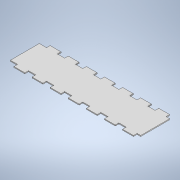
# Autodesk Inventor part: BridgeRoof
Saved by Autodesk Inventor 2022 (Build 260153000, 153)
## iProperties
Created: 2022-03-02
Part Number: BridgeRoof
Material: Generic
Document SubType Name: Modeling
Designer: anjarwala7025
Density: 1 g/cm^3
Appearance: Default
Author: anjarwala7025
Autodesk Inventor part; units mm, degrees
ref_plane "YZ Plane" through (0, 0, 0) normal (1, 0, 0) x (0, 1, 0)
ref_plane "XZ Plane" through (0, 0, 0) normal (0, 1, 0) x (-1, 0, 0)
ref_plane "XY Plane" through (0, 0, 0) normal (0, 0, 1) x (1, 0, 0)
sketch "Sketch1" plane through (0, 0, 0) normal (0, 1, 0) x (-1, 0, 0)
  line L0 (0, 0) -> (-457.2, 0)
  line L1 (-457.2, 0) -> (-457.2, -127)
  line L2 (-457.2, -127) -> (0, -127)
  line L3 (0, -127) -> (0, 0)
  dimension "d0" = 457.2
  dimension "d1" = 127
  constraints: 8 end point, 2 parallel, 1 horizontal, 1 perpendicular
  measures "d0" distance of L2.end L1.end
  measures "d1" distance of L1.end L0.end
extrude "Extrusion1" add sketch "Sketch1" along normal blind 3.175
sketch "Sketch2" plane through (0, 3.175, 0) normal (0, 1, 0) x (1, 0, 0)
  line L0 (0, 127) -> (0, 0) projected
  line L1 (0, 114.3) -> (25.4, 114.3)
  line L2 (25.4, 114.3) -> (25.4, 127)
  line L3 (457.2, 127) -> (0, 127) projected
  line L4 (63.5, 127) -> (63.5, 114.3)
  line L5 (63.5, 114.3) -> (88.9, 114.3)
  line L6 (88.9, 114.3) -> (88.9, 127)
  line L7 (127, 127) -> (127, 114.3)
  line L8 (127, 114.3) -> (152.4, 114.3)
  line L9 (152.4, 114.3) -> (152.4, 127)
  line L10 (190.5, 127) -> (190.5, 114.3)
  line L11 (190.5, 114.3) -> (215.9, 114.3)
  line L12 (215.9, 114.3) -> (215.9, 127)
  line L13 (254, 127) -> (254, 114.3)
  line L14 (254, 114.3) -> (279.4, 114.3)
  line L15 (279.4, 114.3) -> (279.4, 127)
  line L16 (317.5, 127) -> (317.5, 114.3)
  line L17 (317.5, 114.3) -> (342.9, 114.3)
  line L18 (342.9, 114.3) -> (342.9, 127)
  line L19 (381, 127) -> (381, 114.3)
  line L20 (381, 114.3) -> (406.4, 114.3)
  line L21 (406.4, 114.3) -> (406.4, 127)
  line L22 (444.5, 127) -> (444.5, 114.3)
  line L23 (444.5, 114.3) -> (457.2, 114.3)
  line L24 (457.2, 0) -> (457.2, 127) projected
  line L25 (0, 114.3) -> (0, 127)
  line L26 (63.5, 127) -> (88.9, 127)
  line L27 (127, 127) -> (152.4, 127)
  line L28 (190.5, 127) -> (215.9, 127)
  line L29 (254, 127) -> (279.4, 127)
  line L30 (317.5, 127) -> (342.9, 127)
  line L31 (381, 127) -> (406.4, 127)
  line L32 (444.5, 127) -> (457.2, 127)
  line L33 (0, 127) -> (25.4, 127)
  point P0 (457.2, 114.3)
  point P1 (25.4, 127)
  dimension "d4" = 25.4
  dimension "d6" = 12.7
  dimension "d7" = 12.7
  dimension "d8" = 12.7
  dimension "d9" = 25.4
  dimension "d10" = 38.1
  dimension "d11" = 25.4
  dimension "d12" = 38.1
  dimension "d13" = 25.4
  dimension "d14" = 38.1
  dimension "d15" = 25.4
  dimension "d16" = 38.1
  dimension "d17" = 25.4
  dimension "d18" = 38.1
  dimension "d19" = 25.4
  dimension "d20" = 38.1
  dimension "d21" = 12.7
  dimension "d22" = 0
  dimension "d42" = 12.7
  constraints: 62 end point, 13 vertical, 9 perpendicular, 7 horizontal, 1 collinear, 1 point on line, 14 other
  measures "d4" distance of L1.start L1.end
  measures "d7" distance of L1.end L2.end
  measures "d8" distance of L4.start L4.end
  measures "d9" distance of L4.end L5.end
  measures "d10" distance between parallel lines of L4 L2
  measures "d11" distance of L7.end L8.end
  measures "d12" distance between parallel lines of L7 L6
  measures "d13" distance of L10.end L11.end
  measures "d14" distance between parallel lines of L10 L9
  measures "d15" distance of L13.end L14.end
  measures "d16" distance between parallel lines of L13 L12
  measures "d17" distance of L16.end L17.end
  measures "d18" distance between parallel lines of L16 L15
  measures "d19" distance of L19.end L20.end
  measures "d20" distance between parallel lines of L19 L18
  measures "d21" distance of L22.end L23.end
  measures "d22" distance from line of L24 L23.end
  measures "d42" distance of L22.start L22.end
extrude "Extrusion2" cut sketch "Sketch2" against normal through all
sketch "Sketch3" plane through (0, 3.175, 0) normal (0, 1, 0) x (1, 0, 0)
  line L0 (0, 0) -> (457.2, 0) projected
  line L1 (0, 0) -> (25.4, 0)
  line L2 (25.4, 0) -> (25.4, 12.7)
  line L3 (25.4, 12.7) -> (0, 12.7)
  line L4 (0, 12.7) -> (0, 0)
  line L5 (63.5, 0) -> (88.9, 0)
  line L6 (88.9, 0) -> (88.9, 12.7)
  line L7 (88.9, 12.7) -> (63.5, 12.7)
  line L8 (63.5, 12.7) -> (63.5, 0)
  line L9 (127, 0) -> (152.4, 0)
  line L10 (152.4, 0) -> (152.4, 12.7)
  line L11 (152.4, 12.7) -> (127, 12.7)
  line L12 (127, 12.7) -> (127, 0)
  line L13 (190.5, 0) -> (215.9, 0)
  line L14 (215.9, 0) -> (215.9, 12.7)
  line L15 (215.9, 12.7) -> (190.5, 12.7)
  line L16 (190.5, 12.7) -> (190.5, 0)
  line L17 (254, 0) -> (279.4, 0)
  line L18 (279.4, 0) -> (279.4, 12.7)
  line L19 (279.4, 12.7) -> (254, 12.7)
  line L20 (254, 12.7) -> (254, 0)
  line L21 (317.5, 0) -> (342.9, 0)
  line L22 (342.9, 0) -> (342.9, 12.7)
  line L23 (342.9, 12.7) -> (317.5, 12.7)
  line L24 (317.5, 12.7) -> (317.5, 0)
  line L25 (381, 0) -> (406.4, 0)
  line L26 (406.4, 0) -> (406.4, 12.7)
  line L27 (406.4, 12.7) -> (381, 12.7)
  line L28 (381, 12.7) -> (381, 0)
  line L29 (457.2, 0) -> (457.2, 114.3) projected
  line L30 (457.2, 0) -> (444.5, 0)
  line L31 (444.5, 0) -> (444.5, 12.7)
  line L32 (444.5, 12.7) -> (457.2, 12.7)
  line L33 (457.2, 12.7) -> (457.2, 0)
  dimension "d25" = 25.4
  dimension "d26" = 12.7
  dimension "d27" = 25.4
  dimension "d28" = 38.1
  dimension "d29" = 25.4
  dimension "d30" = 25.4
  dimension "d31" = 25.4
  dimension "d32" = 25.4
  dimension "d33" = 25.4
  dimension "d34" = 12.7
  dimension "d35" = 38.1
  dimension "d36" = 38.1
  dimension "d37" = 38.1
  dimension "d38" = 38.1
  dimension "d39" = 38.1
  constraints: 64 end point, 16 parallel, 11 point on line, 8 horizontal, 8 perpendicular
  measures "d25" distance of L3.end L2.end
  measures "d26" distance of L2.end L1.end
  measures "d27" distance of L7.end L6.end
  measures "d28" distance between parallel lines of L8 L2
  measures "d29" distance of L11.end L10.end
  measures "d30" distance of L15.end L14.end
  measures "d31" distance of L19.end L18.end
  measures "d32" distance of L23.end L22.end
  measures "d33" distance of L27.end L26.end
  measures "d34" distance of L31.end L32.end
  measures "d35" distance between parallel lines of L12 L6
  measures "d36" distance between parallel lines of L16 L10
  measures "d37" distance between parallel lines of L20 L14
  measures "d38" distance between parallel lines of L24 L18
  measures "d39" distance between parallel lines of L28 L22
extrude "Extrusion3" cut sketch "Sketch3" against normal through all
body "Solid1"
